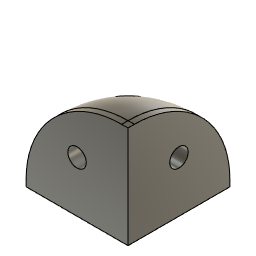
box_joint (Autodesk Fusion 360 design; units mm, degrees)
Autodesk Fusion 360 part; units mm, degrees
sketch "スケッチ1" plane through (0, 0, 0) normal (0, 0, 1) x (1, 0, 0)
  line L0 (-25, 25) -> (25, 25)
  line L1 (25, 25) -> (25, -25)
  line L2 (25, -25) -> (-25, -25)
  line L3 (-25, -25) -> (-25, 25)
  constraint horizontal L0
  constraint vertical L1
  constraint horizontal L2
  constraint vertical L3
extrude "押し出し1" add sketch "スケッチ1" along normal blind 3 makes body 1
move_face "面を移動1" by (70, 0, 0) 1 faces at (-8.3333, 8.3333, 3) on bodies 1
move_face "面を移動2" by (0, 50, 0) 1 faces at (-8.3333, 8.3333, 3) on bodies 1
copy_body "ボディ -> コンポーネント1" bodies 1 removing the originals makes body 2 in component "底面プレート1"
move_face "面を移動1'" by (10, 0, 0) 1 faces at (-8.3333, 8.3333, 3) on bodies 2 in component "底面プレート1"
sketch "スケッチ2" plane through (0, 0, 0) normal (0, 0, 1) x (1, 0, 0)
sketch "スケッチ3" plane through (0, 0, 0) normal (1, 0, 0) x (0, 1, 0)
  line L0 (0, 100) -> (50, 100)
  line L1 (50, 100) -> (50, 50)
  line L2 (50, 50) -> (0, 50)
  line L3 (0, 50) -> (0, 100)
  constraint horizontal L0
  constraint vertical L1
  constraint horizontal L2
  constraint vertical L3
extrude "押し出し2" add sketch "スケッチ3" along normal blind 3 separate body makes body 3
copy_body "ボディ -> コンポーネント2" bodies 3 removing the originals makes body 4 in component "プレート2"
sketch "スケッチ4" plane through (0, 0, 0) normal (0, 1, 0) x (1, 0, 0)
sketch "スケッチ5" plane through (0, 0, 0) normal (1, 0, 0) x (0, 1, 0)
  line L0 (50, 50) -> (100, 50)
  line L1 (100, 50) -> (100, 0)
  line L2 (100, 0) -> (50, 0)
  line L3 (50, 0) -> (50, 50)
  constraint horizontal L0
  constraint vertical L1
  constraint horizontal L2
  constraint vertical L3
extrude "押し出し3" add sketch "スケッチ5" along normal blind 3 separate body makes body 5
copy_body "ボディ -> コンポーネント3" bodies 5 removing the originals makes body 6 in component "プレート3"
sketch "スケッチ6" plane through (0, 0, 0) normal (0, 1, 0) x (1, 0, 0)
  line L0 (40, -42) -> (84, -42)
  line L1 (84, -42) -> (84, 8)
  line L2 (84, 8) -> (40, 8)
  line L3 (40, 8) -> (40, -42)
  constraint horizontal L0
  constraint vertical L1
  constraint horizontal L2
  constraint vertical L3
extrude "押し出し4" add sketch "スケッチ6" along normal blind 3 separate body makes body 7
copy_body "ボディ -> コンポーネント4" bodies 7 removing the originals makes body 8 in component "プレート4"
sketch "スケッチ7" plane through (0, 0, 0) normal (0, 1, 0) x (1, 0, 0)
  line L0 (50, -20) -> (94, -20)
  line L1 (94, -20) -> (94, -70)
  line L2 (94, -70) -> (50, -70)
  line L3 (50, -70) -> (50, -20)
  dimension "d45" = 44
  dimension "d46" = 50
  constraint horizontal L0
  constraint vertical L1
  constraint horizontal L2
  constraint vertical L3
  measures "d45" distance of L0.start L0.end
  measures "d46" distance of L0.start L2.end
extrude "押し出し5" add sketch "スケッチ7" along normal blind 3 separate body makes body 9
copy_body "ボディ -> コンポーネント5" bodies 9 removing the originals makes body 10 in component "プレート5"
sketch "スケッチ8" plane through (0, 0, 0) normal (0, 1, 0) x (1, 0, 0)
sketch "スケッチ9" plane through (0, 0, 0) normal (0, 0, 1) x (1, 0, 0)
  line L0 (50, 25) -> (100, 25)
  line L1 (100, 25) -> (100, -25)
  line L2 (100, -25) -> (50, -25)
  line L3 (50, -25) -> (50, 25)
  constraint horizontal L0
  constraint vertical L1
  constraint horizontal L2
  constraint vertical L3
extrude "押し出し6" add sketch "スケッチ9" along normal blind 3 separate body makes body 11
copy_body "ボディ -> コンポーネント6" bodies 11 removing the originals makes body 12 in component "プレート6"
sketch "スケッチ10" plane through (0, 0, 0) normal (0, 0, 1) x (1, 0, 0)
  line L0 (60, -25) -> (50, -25)
  line L1 (50, -25) -> (50, -15)
  line L2 (50, -15) -> (60, -15)
  line L3 (60, -15) -> (60, -25)
  dimension "d89" = 10
  dimension "d90" = 10
  constraint horizontal L0
  constraint vertical L1
  constraint horizontal L2
  constraint vertical L3
  measures "d89" distance of L1.end L2.end
  measures "d90" distance of L0.start L2.end
extrude "押し出し7" add sketch "スケッチ10" along normal blind 25 separate body makes body 13
sketch "スケッチ11" plane through (0, 0, 25) normal (0, 0, 1) x (-1, 0, 0)
  line L0 (-60, 15) -> (-50, 15)
  line L1 (-50, 15) -> (-50, 25)
  line L2 (-50, 25) -> (-60, 25)
  line L3 (-60, 25) -> (-60, 15)
hole "穴1" at (55, -20, 25) direction (0, 0, -1) diameter 3.9 depth 3.7 tip angle 180 bodies 13
hole "穴2" at (55, -25, 12.5) direction (0, 1, 0) diameter 3.9 depth 3.7 tip angle 180 bodies 13
hole "穴3" at (60, -20, 12.5) direction (-1, 0, 0) diameter 3.9 depth 3.7 tip angle 180 bodies 13
delete_body "RemoveBody8" bodies 13
sketch "スケッチ12" plane through (0, 0, 0) normal (0, 0, 1) x (1, 0, 0)
  line L0 (69, 0) -> (85, 0)
  line L1 (85, 0) -> (85, 16)
  line L2 (85, 16) -> (69, 16)
  line L3 (69, 16) -> (69, 0)
  dimension "d104" = 16
  dimension "d105" = 16
  constraint horizontal L0
  constraint vertical L1
  constraint horizontal L2
  constraint vertical L3
  measures "d104" distance of L1.end L2.end
  measures "d105" distance of L0.end L1.end
extrude "押し出し8" add sketch "スケッチ12" along normal blind 16 separate body makes body 14
fillet "フィレット2" radius 15 3 edges at (69, 16, 8) (69, 8, 16) (77, 16, 16) on bodies 14
hole "穴4" at (77, 0, 8) direction (0, 1, 0) diameter 2.9 depth 18 tip angle 180 bodies 14
hole "穴5" at (85, 8, 8) direction (-1, 0, 0) diameter 2.9 depth 18 tip angle 180 bodies 14
hole "穴6" at (77, 8, 0) direction (0, 0, 1) diameter 2.9 depth 18 tip angle 180 bodies 14
copy_body "ボディ -> コンポーネント8" bodies 14 removing the originals makes body 15 in component "ジョイント"
copy_body "ボディのコピーと貼り付け1" bodies 15 body 15 seen with x (1, 0, 0) y (0, 1, 0) z (0, 0, 1) at (27.0459, 56.3117, -19.3799) makes body 16
move_body "移動1" bodies 16 to x (1, 0, 0) y (0, 1, 0) z (0, 0, 1) at (0, 20, 0)
copy_body "ボディのコピーと貼り付け2" bodies 15 body 15 seen with x (1, 0, 0) y (0, 1, 0) z (0, 0, 1) at (27.0459, 56.3117, -19.3799) makes body 17
move_body "移動2" bodies 17 to x (1, 0, 0) y (0, 1, 0) z (0, 0, 1) at (20, 0, 0)
copy_body "ボディのコピーと貼り付け3" bodies 15 body 15 seen with x (1, 0, 0) y (0, 1, 0) z (0, 0, 1) at (27.0459, 56.3117, -19.3799) makes body 18
move_body "移動3" bodies 18 to x (1, 0, 0) y (0, 1, 0) z (0, 0, 1) at (0, 0, 20)
copy_body "ボディ -> コンポーネント9" bodies 16 removing the originals makes body 19 in component "ジョイント6"
copy_body "ボディ -> コンポーネント10" bodies 18 removing the originals makes body 20 in component "ジョイント7"
copy_body "ボディ -> コンポーネント11" bodies 17 removing the originals makes body 21 in component "ジョイント9"
move_face "面を移動1''" to x (0, 1, 0) y (-1, 0, 0) z (0, 0, 1) at (189.3575, -34.7342, 0) 1 faces at (112.0459, 78.4964, -11.3438) on bodies 19 in component "ジョイント6"
hole "穴1'" at (0, 41, 94) direction (1, 0, 0) diameter 3.2 depth 3 tip angle 180 bodies 4 in component "プレート2"
hole "穴2'" at (0, 9, 94) direction (1, 0, 0) diameter 3.2 depth 3 tip angle 180 bodies 4 in component "プレート2"
hole "穴3'" at (0, 9, 56) direction (1, 0, 0) diameter 3.2 depth 3 tip angle 180 bodies 4 in component "プレート2"
hole "穴4'" at (0, 41, 56) direction (1, 0, 0) diameter 3.2 depth 3 tip angle 180 bodies 4 in component "プレート2"
hole "穴1''" at (56, 3, 64) direction (0, -1, 0) diameter 3.2 depth 3 tip angle 180 bodies 10 in component "プレート5"
hole "穴2''" at (88, 3, 64) direction (0, -1, 0) diameter 3.2 depth 3 tip angle 180 bodies 10 in component "プレート5"
hole "穴3''" at (56, 3, 26) direction (0, -1, 0) diameter 3.2 depth 3 tip angle 180 bodies 10 in component "プレート5"
hole "穴4''" at (88, 3, 26) direction (0, -1, 0) diameter 3.2 depth 3 tip angle 180 bodies 10 in component "プレート5"
hole "穴1'''" at (3, 91, 44) direction (-1, 0, 0) diameter 3.2 depth 3 tip angle 180 bodies 6 in component "プレート3"
hole "穴2'''" at (3, 59, 44) direction (-1, 0, 0) diameter 3.2 depth 3 tip angle 180 bodies 6 in component "プレート3"
hole "穴3'''" at (3, 59, 6) direction (-1, 0, 0) diameter 3.2 depth 3 tip angle 180 bodies 6 in component "プレート3"
hole "穴4'''" at (3, 91, 6) direction (-1, 0, 0) diameter 3.2 depth 3 tip angle 180 bodies 6 in component "プレート3"
hole "穴1''''" at (46, 0, 36) direction (0, 1, 0) diameter 3.2 depth 3 tip angle 180 bodies 8 in component "プレート4"
hole "穴2''''" at (78, 0, 36) direction (0, 1, 0) diameter 3.2 depth 3 tip angle 180 bodies 8 in component "プレート4"
hole "穴3''''" at (46, 0, -2) direction (0, 1, 0) diameter 3.2 depth 3 tip angle 180 bodies 8 in component "プレート4"
hole "穴4''''" at (78, 0, -2) direction (0, 1, 0) diameter 3.2 depth 3 tip angle 180 bodies 8 in component "プレート4"
hole "穴1'''''" at (-16, -16, 0) direction (0, 0, 1) diameter 3.2 depth 3 tip angle 180 bodies 2 in component "底面プレート1"
hole "穴2'''''" at (-16, 16, 0) direction (0, 0, 1) diameter 3.2 depth 3 tip angle 180 bodies 2 in component "底面プレート1"
hole "穴3'''''" at (16, -16, 0) direction (0, 0, 1) diameter 3.2 depth 3 tip angle 180 bodies 2 in component "底面プレート1"
hole "穴4'''''" at (16, 16, 0) direction (0, 0, 1) diameter 3.2 depth 3 tip angle 180 bodies 2 in component "底面プレート1"
hole "穴1''''''" at (59, 16, 3) direction (0, 0, -1) diameter 3.2 depth 3 tip angle 180 bodies 12 in component "プレート6"
hole "穴2''''''" at (59, -16, 3) direction (0, 0, -1) diameter 3.2 depth 3 tip angle 180 bodies 12 in component "プレート6"
hole "穴3''''''" at (91, 16, 3) direction (0, 0, -1) diameter 3.2 depth 3 tip angle 180 bodies 12 in component "プレート6"
hole "穴4''''''" [suppressed] in component "プレート6"
component "底面プレート1" placed x (1, 0, 0) y (0, 1, 0) z (0, 0, 1) at (5.9791, 10.285, 3.2571)
component "プレート2" placed x (1, 0, 0) y (0, 1, 0) z (0, 0, 1) at (-19.0209, -14.715, -43.7429)
component "プレート3" placed x (1, 0, 0) y (0, 1, 0) z (0, 0, 1) at (27.9791, -64.715, 6.2571)
component "プレート4" placed x (1, 0, 0) y (0, 1, 0) z (0, 0, 1) at (-56.0209, -14.715, 14.2571)
component "プレート5" placed x (1, 0, 0) y (0, 1, 0) z (0, 0, 1) at (-66.0209, 32.285, -13.7429)
component "プレート6" placed x (1, 0, 0) y (0, 1, 0) z (0, 0, 1) at (-69.0209, 10.285, 56.2571)
component "ジョイント" placed x (1, 0, 0) y (0, 1, 0) z (0, 0, 1) at (-57.0209, -11.715, 6.2571)
component "ジョイント" placed x (0, 1, 0) y (-1, 0, 0) z (0, 0, 1) at (27.9791, -52.715, 6.2571)
component "ジョイント" placed x (-1, 0, 0) y (0, -1, 0) z (0, 0, 1) at (68.9791, 32.285, 6.2571)
component "ジョイント" placed x (0, -1, 0) y (1, 0, 0) z (0, 0, 1) at (-16.0209, 73.285, 6.2571)
component "ジョイント6" placed x (-1, 0, 0) y (0, 1, 0) z (0, 0, -1) at (96.025, -88.0267, 36.8772)
component "ジョイント7" placed x (0, 1, 0) y (1, 0, 0) z (0, 0, -1) at (-72.3326, -79.7609, 56.8772)
component "ジョイント9" placed x (1, 0, 0) y (0, -1, 0) z (0, 0, -1) at (-104.0668, 88.5967, 36.8772)
component "ジョイント9" placed x (0, -1, 0) y (-1, 0, 0) z (0, 0, -1) at (84.2908, 120.3309, 36.8772)
